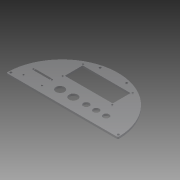
# Autodesk Inventor part: Top Plate
Saved by Autodesk Inventor 2015 (Build 190159000, 159)
## iProperties
Created: 2015-10-10
Part Number: Top Plate
Material: Acrylic
Document SubType Name: Modeling
Designer: James
Density: 1.188 g/cm^3
Appearance: Transparent - Clear
Mass: 39.7763 g
Surface Area: 237.425 cm^2
Volume: 33.4818 cm^3
Author: James
Autodesk Inventor part; units mm, degrees
ref_plane "YZ Plane" through (0, 0, 0) normal (1, 0, 0) x (0, 1, 0)
ref_plane "XZ Plane" through (0, 0, 0) normal (0, 1, 0) x (-1, 0, 0)
ref_plane "XY Plane" through (0, 0, 0) normal (0, 0, 1) x (1, 0, 0)
sketch "Sketch1" plane through (0, 0, 0) normal (0, 1, 0) x (-1, 0, 0)
  circle A0 centre (0, 20) radius 1.65
  circle A1 centre (0, -20) radius 1.65
  line L0 (77.6306, -82.403) -> (77.6306, 82.403)
  arc A2 (75.5821, 84.4024) -> (75.5821, -84.4024) centre (77.6306, 0) ccw
  arc A3 (75.5821, -84.4024) -> (77.6306, -82.403) centre (75.6306, -82.403) ccw
  arc A4 (77.6306, 82.403) -> (75.5821, 84.4024) centre (75.6306, 82.403) ccw
  circle A5 centre (73.783, 81.2341) radius 1.65
  circle A6 centre (73.783, -81.2341) radius 1.65
  arc A7 (75.5821, -84.4024) -> (77.6306, -82.403) centre (75.6306, -82.403) ccw
  arc A8 (75.5821, 84.4024) -> (75.5821, -84.4024) centre (77.6306, 0) ccw
  arc A9 (77.6306, 82.403) -> (75.5821, 84.4024) centre (75.6306, 82.403) ccw
  line L1 (77.6306, 82.403) -> (77.6306, -82.403)
  circle A10 centre (73.783, -81.2341) radius 1.65
  circle A11 centre (73.783, 81.2341) radius 1.65
  circle A12 centre (0, -20) radius 1.65
  circle A13 centre (0, 20) radius 1.65
  arc A14 (75.5821, -84.4024) -> (77.6306, -82.403) centre (75.6306, -82.403) ccw
  arc A15 (75.5821, 84.4024) -> (75.5821, -84.4024) centre (77.6306, 0) ccw
  arc A16 (77.6306, 82.403) -> (75.5821, 84.4024) centre (75.6306, 82.403) ccw
  line L2 (77.6306, 82.403) -> (77.6306, -82.403)
  circle A17 centre (73.783, -81.2341) radius 1.65
  circle A18 centre (73.783, 81.2341) radius 1.65
  circle A19 centre (0, -20) radius 1.65
  circle A20 centre (0, 20) radius 1.65
  arc A21 (75.5821, -84.4024) -> (77.6306, -82.403) centre (75.6306, -82.403) ccw
  arc A22 (75.5821, 84.4024) -> (75.5821, -84.4024) centre (77.6306, 0) ccw
  arc A23 (77.6306, 82.403) -> (75.5821, 84.4024) centre (75.6306, 82.403) ccw
  line L3 (77.6306, 82.403) -> (77.6306, -82.403)
  circle A24 centre (73.783, -81.2341) radius 1.65
  circle A25 centre (73.783, 81.2341) radius 1.65
  circle A26 centre (0, -20) radius 1.65
  circle A27 centre (0, 20) radius 1.65
  line L4 (52.2117, -66.85) -> (50.7117, -66.85)
  line L5 (50.7117, -66.85) -> (50.7117, -42.45)
  line L6 (50.7117, -42.45) -> (52.2117, -42.45)
  line L7 (52.2117, -42.45) -> (53.7117, -42.45)
  line L8 (53.7117, -42.45) -> (53.7117, -66.85)
  line L9 (53.7117, -66.85) -> (52.2117, -66.85)
  circle A28 centre (52.2117, -68.65) radius 1.25
  circle A29 centre (67.2117, -68.65) radius 1.25
  circle A30 centre (52.2117, -40.65) radius 1.25
  circle A31 centre (67.2117, -40.65) radius 1.25
  arc A32 (75.5821, -84.4024) -> (77.6306, -82.403) centre (75.6306, -82.403) ccw
  arc A33 (75.5821, 84.4024) -> (75.5821, -84.4024) centre (77.6306, 0) ccw
  arc A34 (77.6306, 82.403) -> (75.5821, 84.4024) centre (75.6306, 82.403) ccw
  line L10 (77.6306, 82.403) -> (77.6306, -82.403)
  circle A35 centre (73.783, -81.2341) radius 1.65
  circle A36 centre (73.783, 81.2341) radius 1.65
  circle A37 centre (0, -20) radius 1.65
  circle A38 centre (0, 20) radius 1.65
  circle A39 centre (39.2929, 37.5) radius 1.25
  circle A40 centre (8.2929, 37.5) radius 1.25
  circle A41 centre (39.2929, -37.5) radius 1.25
  circle A42 centre (8.2929, -37.5) radius 1.25
  line L11 (37.2929, 36.15) -> (10.2929, 36.15)
  line L12 (10.2929, 36.15) -> (10.2929, -36.15)
  line L13 (10.2929, -36.15) -> (37.2929, -36.15)
  line L14 (37.2929, -36.15) -> (37.2929, 36.15)
  line L15 (52.2117, -66.85) -> (50.7117, -66.85)
  line L16 (50.7117, -66.85) -> (50.7117, -42.45)
  line L17 (50.7117, -42.45) -> (52.2117, -42.45)
  line L18 (52.2117, -42.45) -> (53.7117, -42.45)
  line L19 (53.7117, -42.45) -> (53.7117, -66.85)
  line L20 (53.7117, -66.85) -> (52.2117, -66.85)
  circle A43 centre (52.2117, -68.65) radius 1.25
  circle A44 centre (67.2117, -68.65) radius 1.25
  circle A45 centre (52.2117, -40.65) radius 1.25
  circle A46 centre (67.2117, -40.65) radius 1.25
  arc A47 (75.5821, -84.4024) -> (77.6306, -82.403) centre (75.6306, -82.403) ccw
  arc A48 (75.5821, 84.4024) -> (75.5821, -84.4024) centre (77.6306, 0) ccw
  arc A49 (77.6306, 82.403) -> (75.5821, 84.4024) centre (75.6306, 82.403) ccw
  line L21 (77.6306, 82.403) -> (77.6306, -82.403)
  circle A50 centre (73.783, -81.2341) radius 1.65
  circle A51 centre (73.783, 81.2341) radius 1.65
  circle A52 centre (0, -20) radius 1.65
  circle A53 centre (0, 20) radius 1.65
  circle A54 centre (39.2929, 37.5) radius 1.25
  circle A55 centre (8.2929, 37.5) radius 1.25
  circle A56 centre (39.2929, -37.5) radius 1.25
  circle A57 centre (8.2929, -37.5) radius 1.25
  line L22 (37.2929, 36.15) -> (10.2929, 36.15)
  line L23 (10.2929, 36.15) -> (10.2929, -36.15)
  line L24 (10.2929, -36.15) -> (37.2929, -36.15)
  line L25 (37.2929, -36.15) -> (37.2929, 36.15)
  circle A58 centre (58.783, -1.7659) radius 6.5
  circle A59 centre (58.783, 47.8112) radius 4.5
  circle A60 centre (58.783, 32.8112) radius 4.5
  circle A61 centre (58.783, 17.8112) radius 4.5
  circle A62 centre (58.783, -21.7659) radius 6.5
  line L26 (52.2117, -66.85) -> (50.7117, -66.85)
  line L27 (50.7117, -66.85) -> (50.7117, -42.45)
  line L28 (50.7117, -42.45) -> (52.2117, -42.45)
  line L29 (52.2117, -42.45) -> (53.7117, -42.45)
  line L30 (53.7117, -42.45) -> (53.7117, -66.85)
  line L31 (53.7117, -66.85) -> (52.2117, -66.85)
  circle A63 centre (52.2117, -68.65) radius 1.25
  circle A64 centre (67.2117, -68.65) radius 1.25
  circle A65 centre (52.2117, -40.65) radius 1.25
  circle A66 centre (67.2117, -40.65) radius 1.25
  point P0 (0, 0)
  dimension "d1" = 3.3
  dimension "d3" = 3.3
  dimension "d11" = 2
  dimension "d16" = 3.3
  dimension "d17" = 3.3
  constraints: 67 centre point, 64 end point, 36 point on circle, 4 tangent, 1 equal radius, 1 midpoint, 1 vertical
  measures "d1" diameter of A0
  measures "d3" diameter of A1
  measures "d11" radius of A3
  measures "d16" diameter of A5
  measures "d17" diameter of A6
extrude "Extrusion6" add sketch "Sketch1" along normal blind 3
body "Solid5"
